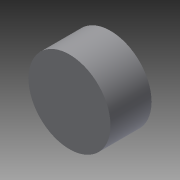
# Autodesk Inventor part: Rad
Saved by Autodesk Inventor 2014 (Build 180170000, 170)
## iProperties
Created: 2015-11-28
Part Number: Rad
Material: Generisch
Document SubType Name: Modeling
Designer: nrk
Density: 1 g/cm^3
Appearance: Vorgabe
Author: nrk
Autodesk Inventor part; units mm, degrees
ref_plane "YZ Plane" through (0, 0, 0) normal (1, 0, 0) x (0, 1, 0)
ref_plane "XZ Plane" through (0, 0, 0) normal (0, 1, 0) x (-1, 0, 0)
ref_plane "XY Plane" through (0, 0, 0) normal (0, 0, 1) x (1, 0, 0)
sketch "Skizze1" plane through (0, 0, 0) normal (0, 1, 0) x (-1, 0, 0)
  circle A0 centre (0, 0) radius 50
  dimension "d0" = 100
  constraints: 1 centre point, 1 coincident
  measures "d0" diameter of A0
extrude "Extrusion1" add sketch "Skizze1" along normal blind 50
